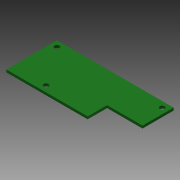
# Autodesk Inventor part: InjectorBoard
Saved by Autodesk Inventor 2014 (Build 180170000, 170)
## iProperties
Created: 2015-01-07
Part Number: InjectorBoard
Material: Generic
Document SubType Name: Modeling
Designer: Owner
Density: 1 g/cm^3
Appearance: Smooth - Dark Forest Green
Author: Owner
Autodesk Inventor part; units mm, degrees
ref_plane "YZ Plane" through (0, 0, 0) normal (1, 0, 0) x (0, 1, 0)
ref_plane "XZ Plane" through (0, 0, 0) normal (0, 1, 0) x (-1, 0, 0)
ref_plane "XY Plane" through (0, 0, 0) normal (0, 0, 1) x (1, 0, 0)
sketch "Sketch1" plane through (0, 0, 0) normal (0, 1, 0) x (-1, 0, 0)
  line L0 (-33.6146, 10.7635) -> (42.5854, 10.7635)
  line L1 (42.5854, 10.7635) -> (42.5854, -22.2565)
  line L2 (42.5854, -22.2565) -> (-33.6146, -22.2565)
  line L3 (-33.6146, -22.2565) -> (-33.6146, 10.7635)
  line L4 (-33.6146, -22.2565) -> (-10.7151, -22.2565)
  line L5 (-33.6146, -8.8905) -> (-33.6146, -22.2565)
  line L6 (-33.6146, 10.7635) -> (-1.8646, 10.7635)
  line L7 (-1.8646, 10.7635) -> (-1.8646, -1.9365)
  line L8 (-1.8646, -1.9365) -> (-33.6146, -1.9365)
  line L9 (-33.6146, -1.9365) -> (-33.6146, 10.7635)
  point P0 (0, 0)
  dimension "d0" = 76.2
  dimension "d1" = 33.02
  dimension "d37" = 12.7
  dimension "d50" = 31.75
  constraints: 20 end point, 4 parallel, 3 horizontal, 2 perpendicular
  measures "d0" distance of L0.start L0.end
  measures "d1" distance of L2.end L0.start
  measures "d37" distance of L6.end L7.end
  measures "d50" distance of L7.end L8.end
extrude "Extrusion1" add sketch "Sketch1" along normal blind 1.65 contours L0 L1 L2 L3 L8 L7
sketch "Sketch6" plane through (0, 1.65, 0) normal (0, 1, 0) x (1, 0, 0)
  line L0 (33.6146, 1.9365) -> (33.6146, 22.2565) projected
  line L1 (33.6146, 22.2565) -> (-42.5854, 22.2565) projected
  line L2 (-42.5854, 22.2565) -> (-42.5854, -10.7635) projected
  line L3 (-42.5854, -10.7635) -> (1.8646, -10.7635) projected
  circle A0 centre (-38.8262, 18.51) radius 1.5875
  circle A1 centre (29.8554, 18.51) radius 1.5875
  circle A2 centre (-20.6779, -6.763) radius 1.5875
  point P0 (0, 0)
  dimension "d39" = 3.175
  dimension "d40" = 3.175
  dimension "d41" = 3.175
  dimension "d42" = 21.9075
  dimension "d43" = 4.0005
  dimension "d44" = 3.7465
  dimension "d45" = 3.7465
  dimension "d46" = 3.7592
  dimension "d47" = 3.7592
  constraints: 3 centre point
  measures "d39" diameter of A2
  measures "d40" diameter of A0
  measures "d41" diameter of A1
  measures "d42" distance from line of L2 A2.centre
  measures "d43" distance from line of L3 A2.centre
  measures "d44" distance from line of L1 A0.centre
  measures "d45" distance from line of L1 A1.centre
  measures "d46" distance from line of L0 A1.centre
  measures "d47" distance from line of L2 A0.centre
extrude "Extrusion6" cut sketch "Sketch6" against normal blind 7.53
body "Solid1"
